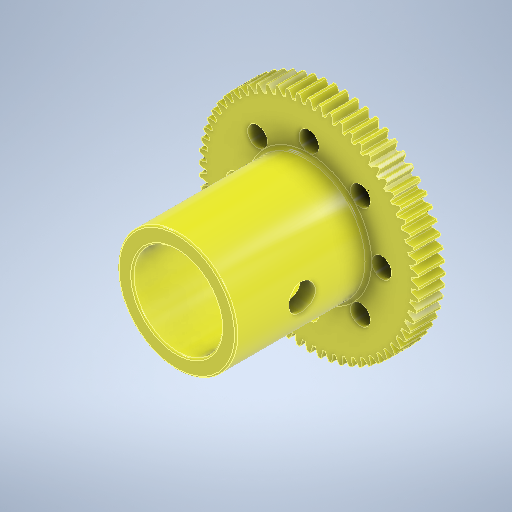
# Autodesk Inventor part: Steering Gear
Saved by Autodesk Inventor 2025.2 (Build 292293000, 293)
## iProperties
CustomPartVersion: 1
Created: 2025-02-06
Part Number: Steering Gear
Material: Steel
Document SubType Name: Modeling
Designer: eason
Categories: <?xml version="1.0" encoding="UTF-16"?> <MemberInstance><Categories><FamilyTemplate><FamilyTemplateParameter ValueType="xs:double" Id="1" ObjectReferenceKey="da_z" ObjectType="kUserParameterObject"/><FamilyTemplateParameter ValueType="xs:double" Id="2" ObjectReferenceKey="da_b" ObjectType="kUserParameterObject"/><FamilyTemplateParameter ValueType="xs:double" Id="3" ObjectReferenceKey="da_beta" ObjectType="kUserParameterObject"/><FamilyTemplateParameter ValueType="xs:double" Id="4" ObjectReferenceKey="da_da" ObjectType="kUserParameterObject"/><FamilyTemplateParameter ValueType="xs:double" Id="5" ObjectReferenceKey="da_aw" ObjectType="kUserParameterObject"/><FamilyTemplateParameter ValueType="xs:string" Id="6" ObjectReferenceKey="EAIAABAAAACIAQAAAAAAAIAAAAAAAAAA" ObjectType="83910656" SubObjectId="SurfaceGeometry"/></FamilyTemplate><ParamToTemplateMap><ParamToTemplate CategoryParameter="//CategoryParameter[@InternalName='046C89C9-8512-4d59-83FE-43B91F4F132A']" TemplateParameter="1"/><ParamToTemplate CategoryParameter="//CategoryParameter[@InternalName='2552DF32-E462-4b46-AEBF-C6C7768E72AC']" TemplateParameter="2"/><ParamToTemplate CategoryParameter="//CategoryParameter[@InternalName='C9EE641D-15FC-4fae-A226-E94C4372FDD7']" TemplateParameter="3"/><ParamToTemplate><ParamToTemplate CategoryParameter="//CategoryParameter[@InternalName='00B6519A-459B-49c7-AD84-2E56D39A5744']" ConstantValue="0.218033"/></ParamToTemplate><ParamToTemplate><ParamToTemplate CategoryParameter="//CategoryParameter[@InternalName='04B31F0E-C7A6-4894-AA32-9629BEFACF47']" ConstantValue="1.000000"/></ParamToTemplate><ParamToTemplate><ParamToTemplate CategoryParameter="//CategoryParameter[@InternalName='43CBEC2E-7847-49e7-A936-2F7889FCB2D9']" ConstantValue="0.250000"/></ParamToTemplate><ParamToTemplate><ParamToTemplate CategoryParameter="//CategoryParameter[@InternalName='B1EFC894-105D-4ebd-86BF-FA20ED196853']" ConstantValue="0.350000"/></ParamToTemplate><ParamToTemplate><ParamToTemplate CategoryParameter="//CategoryParameter[@InternalName='51175063-3D10-4879-93E8-6246FE8B403D']" ConstantValue="2060000000.000000"/></ParamToTemplate><ParamToTemplate><ParamToTemplate CategoryParameter="//CategoryParameter[@InternalName='A3A52E27-4454-46a9-B0BD-C932399B70AF']" ConstantValue="0.300000"/></ParamToTemplate><ParamToTemplate><ParamToTemplate CategoryParameter="//CategoryParameter[@InternalName='91B76062-C214-41d9-B1B9-14D2AB99603D']" ConstantValue="0.100000"/></ParamToTemplate><ParamToTemplate><ParamToTemplate CategoryParameter="//CategoryParameter[@InternalName='374E806E-8B8A-4dda-A9AA-1039D6500AD2']" ConstantValue="10.000000"/></ParamToTemplate><ParamToTemplate><ParamToTemplate CategoryParameter="//CategoryParameter[@InternalName='2D373A89-B862-43d6-8D0B-0CBF12AB9F6C']" ConstantValue="0.349066"/></ParamToTemplate><ParamToTemplate CategoryParameter="//CategoryParameter[@InternalName='37777632-D6A2-4fac-9D53-DB8ACD95C989']" TemplateParameter="4"/><ParamToTemplate CategoryParameter="//CategoryParameter[@InternalName='FD1017F1-B727-4f7e-9707-0F86F1FF9423']" TemplateParameter="5"/><ParamToTemplate><ParamToTemplate CategoryParameter="//CategoryParameter[@InternalName='9E1B4470-B2D3-4ff1-B813-535BB4CDF51A']" ConstantValue="3520000.000000"/></ParamToTemplate><ParamToTemplate><ParamToTemplate CategoryParameter="//CategoryParameter[@InternalName='F8452263-BFF6-458c-9FB1-07C4B99E95CD']" ConstantValue="11400000.000000"/></ParamToTemplate><ParamToTemplate><ParamToTemplate CategoryParameter="//CategoryParameter[@InternalName='3E3BB259-FD49-497f-8171-6EBC954A3479']" ConstantValue="2.000000"/></ParamToTemplate><ParamToTemplate CategoryParameter="//CategoryParameter[@InternalName='27C3BAF2-7550-4e4b-AE2C-0DB134B7D9B7']" TemplateParameter="6"/></ParamToTemplateMap><Category DisplayName="Gear" InternalName="DC85795E-93AB-48d5-8EEE-5A27447B64BD" Mnemonic="Gear"><CategoryParameter DisplayName="z" InternalName="046C89C9-8512-4d59-83FE-43B91F4F132A" Mnemonic="z"/><CategoryParameter DisplayName="b" InternalName="2552DF32-E462-4b46-AEBF-C6C7768E72AC" Mnemonic="b"/><CategoryParameter DisplayName="||b|" InternalName="C9EE641D-15FC-4fae-A226-E94C4372FDD7" Mnemonic="beta"/><CategoryParameter DisplayName="x" InternalName="00B6519A-459B-49c7-AD84-2E56D39A5744" Mnemonic="x"/><CategoryParameter DisplayName="a*" InternalName="04B31F0E-C7A6-4894-AA32-9629BEFACF47" Mnemonic="a"/><CategoryParameter DisplayName="c*" InternalName="43CBEC2E-7847-49e7-A936-2F7889FCB2D9" Mnemonic="c"/><CategoryParameter DisplayName="r|.f|*" InternalName="B1EFC894-105D-4ebd-86BF-FA20ED196853" Mnemonic="rf"/><CategoryParameter DisplayName="E" InternalName="51175063-3D10-4879-93E8-6246FE8B403D" Mnemonic="E"/><CategoryParameter DisplayName="||m|" InternalName="A3A52E27-4454-46a9-B0BD-C932399B70AF" Mnemonic="mi"/><Category DisplayName="SpurGear" InternalName="26C5A22E-A91E-4dfd-A3B3-23CCAFAE1764" Mnemonic="SpurGear"><CategoryParameter DisplayName="m" InternalName="91B76062-C214-41d9-B1B9-14D2AB99603D" Mnemonic="m"/><CategoryParameter DisplayName="P" InternalName="374E806E-8B8A-4dda-A9AA-1039D6500AD2" Mnemonic="PP"/><CategoryParameter DisplayName="||a|" InternalName="2D373A89-B862-43d6-8D0B-0CBF12AB9F6C" Mnemonic="alpha"/><CategoryParameter DisplayName="d|.a|" InternalName="37777632-D6A2-4fac-9D53-DB8ACD95C989" Mnemonic="da"/><CategoryParameter DisplayName="a|.w|" InternalName="FD1017F1-B727-4f7e-9707-0F86F1FF9423" Mnemonic="aw"/><CategoryParameter DisplayName="||s||.Flim|" InternalName="9E1B4470-B2D3-4ff1-B813-535BB4CDF51A" Mnemonic="sFlim"/><CategoryParameter DisplayName="||s||.Hlim|" InternalName="F8452263-BFF6-458c-9FB1-07C4B99E95CD" Mnemonic="sHlim"/><CategoryParameter DisplayName="type" InternalName="3E3BB259-FD49-497f-8171-6EBC954A3479" Mnemonic="type"/><CategoryParameter DisplayName="PitchDiameter" InternalName="27C3BAF2-7550-4e4b-AE2C-0DB134B7D9B7" Mnemonic="IDS_PITCHDIAM"/></Category></Category></Categories></MemberInstance>
Density: 1 g/cm^3
Appearance: Yellow
Author: eason
Autodesk Inventor part; units mm, degrees
sketch "Sketch1" plane through (0, 0, 0) normal (0, 0, 1) x (1, 0, 0)
  circle A0 centre (0, 0) radius 33.2138
  dimension "d0" = 66.4276
  constraints: 1 centre point
  measures "d0" diameter of A0
extrude "Extrusion1" add sketch "Sketch1" along normal blind 8
ref_plane "Work Plane2" through (0, 0, 4) normal (0, 0, 1) x (1, 0, 0)
sketch "Sketch2" plane through (0, 0, 0) normal (0, 0, -1) x (-1, 0, 0)
  circle A0 centre (0, 0) radius 33.2138 projected
  circle A1 centre (0, 0) radius 32
  dimension "d3" = 64
  constraints: 1 centre point, 1 coincident
  measures "d3" diameter of A1
surface extrude "Pitch Diameter" sketch "Sketch2" against normal through all shown no curves A1
ref_plane "Work Plane8" through (0, 0, 0) normal (0.9987955, 0.0490677, 0) x (0, 0, 1)
ref_plane "Work Plane9" through (0, 0, 0) normal (1, 0, 0) x (0, 1, 0)
spur gear teeth "Spur Gear" teeth 64 pitch diameter 64 tip diameter 66.4276 root diameter 61.9361 face width 8 start plane through (0, 0, 0) normal (0, 0, -1) x (-1, 0, 0)
sketch "Sketch3" plane through (0, 0, 8) normal (0, 0, 1) x (1, 0, 0)
  circle A0 centre (0, 0) radius 18
  circle A1 centre (0, 0) radius 13.4
  circle A2 centre (0, 0) radius 3
  dimension "d49" = 36
  dimension "d50" = 26.8
  dimension "d51" = 6
  constraints: 3 centre point, 3 coincident
  measures "d49" diameter of A0
  measures "d50" diameter of A1
  measures "d51" diameter of A2
extrude "Extrusion3" add sketch "Sketch3" along normal blind 40 contours A0
ref_plane "Work Plane11" through (18, 0, 8) normal (1, 0, 0) x (0, 1, 0)
sketch "Sketch4" plane through (18, 0, 8) normal (1, 0, 0) x (0, 1, 0)
  circle A0 centre (0, 20) radius 4
  line L0 (0, -17.6) -> (0, 49.6) projected
  line L1 (18, 40) -> (-18, 40) projected
  point P0 (0, -8)
  dimension "d56" = 8
  dimension "d57" = 20
  constraints: 1 centre point, 1 point on line
  measures "d56" diameter of A0
  measures "d57" distance from line of L1 A0.centre
extrude "Extrusion4" cut sketch "Sketch4" against normal through all
fillet "Fillet1" radius 0.5 2 edges at (-13.4, 0, 48) (-18, 0, 48)
fillet "Fillet2" radius 1 1 edges at (-18, 0, 8)
sketch "Sketch9" plane through (0, 0, 0) normal (0, 0, -1) x (-1, 0, 0)
  circle A0 centre (0, 0) radius 2 construction
  circle A1 centre (0, 0) radius 5
  circle A2 centre (-3.5, 0) radius 1.5
  line L0 (46.4993, 0) -> (-46.4993, 0) projected
  circle A3 centre (0, -3.5) radius 1.5
  circle A4 centre (3.5, 0) radius 1.5
  circle A5 centre (0, 3.5) radius 1.5
  line L1 (3.5, -1.5) -> (2, -1.5)
  line L2 (1.5, -3.5) -> (1.5, -2)
  arc A6 (2, -1.5) -> (1.5, -2) centre (2, -2) ccw
  line L3 (3.5, 1.5) -> (2, 1.5)
  arc A7 (1.5, 2) -> (2, 1.5) centre (2, 2) ccw
  line L4 (1.5, 3.5) -> (1.5, 2)
  line L5 (-1.5, 3.5) -> (-1.5, 2)
  arc A8 (-2, 1.5) -> (-1.5, 2) centre (-2, 2) ccw
  line L6 (-3.5, 1.5) -> (-2, 1.5)
  line L7 (-3.5, -1.5) -> (-2, -1.5)
  arc A9 (-1.5, -2) -> (-2, -1.5) centre (-2, -2) ccw
  line L8 (-1.5, -3.5) -> (-1.5, -2)
  point P0 (1.5, 3.5)
  dimension "d91" = 10
  dimension "d99" = 360
  dimension "d118" = 3
  dimension "d119" = 0.5
  dimension "d122" = 360
  constraints: 16 end point, 8 centre point, 8 point on circle, 4 tangent, 2 coincident, 2 horizontal, 1 perpendicular, 1 point on line, 1 vertical, 48 other
  measures "d91" diameter of A1
  measures "d118" radial gap between concentric circles of A1 A0
  measures "d119" radius of A6
extrude "Extrusion9" cut sketch "Sketch9" against normal up to surface (8 mm away) contours A4 L0 | L0 A4 | A5 | A3 | A4 L1 A6 L2 A3 L8 A9 L7 A2 L0 | L0 A2 L6 A8 L5 A5 L4 A7 L3 A4 | L0 A2 | A2 L0
sketch "Sketch11" plane through (0, 0, 0) normal (0, 0, -1) x (-1, 0, 0)
  circle A0 centre (0, 0) radius 19 projected
  circle A1 centre (0, 0) radius 25
  circle A2 centre (0, -22) radius 3
  line L0 (0, -46.4993) -> (0, 46.4993) projected
  circle A3 centre (15.5563, -15.5563) radius 3
  circle A4 centre (22, 0) radius 3
  circle A5 centre (15.5563, 15.5563) radius 3
  circle A6 centre (0, 22) radius 3
  circle A7 centre (-15.5563, 15.5563) radius 3
  circle A8 centre (-22, 0) radius 3
  circle A9 centre (-15.5563, -15.5563) radius 3
  dimension "d111" = 6
  dimension "d114" = 360
  constraints: 9 centre point, 2 tangent, 1 coincident, 1 point on line, 17 other
  measures "d111" radial gap between concentric circles of A0 A1
extrude "Extrusion11" cut sketch "Sketch11" against normal up to surface (8 mm away) contours A4 | A5 | A3 | A6 L0 | L0 A6 | L0 A2 | A2 L0 | A7 | A9 | A8
fillet "Fillet5" radius 0.5 32 edges at (1.6464, 1.6464, 8) (2.75, 1.5, 8) (5, 0, 8) (2.75, -1.5, 8) (1.6464, -1.6464, 8) (1.5, -2.75, 8) (0, -5, 8) (-1.5, -2.75, 8) (-1.6464, -1.6464, 8) (-2.75, -1.5, 8) (-5, 0, 8) (-2.75, 1.5, 8) (-1.6464, 1.6464, 8) (-1.5, 2.75, 8) (0, 5, 8) (1.5, 2.75, 8) (0, 5, 0) (-1.5, 2.75, 0) (-1.6464, 1.6464, 0) (-2.75, 1.5, 0) (-5, 0, 0) (-2.75, -1.5, 0) (-1.6464, -1.6464, 0) (-1.5, -2.75, 0) (0, -5, 0) (1.5, -2.75, 0) (1.6464, -1.6464, 0) (2.75, -1.5, 0) (5, 0, 0) (2.75, 1.5, 0) (1.6464, 1.6464, 0) (1.5, 2.75, 0)
equation "\"d0\" = da_da"
equation "\"d1\" = da_b"
equation "\"d3\" = da_d"
equation "\"d16\" = da_aw"
equation "\"d43\" = da_aw"
equation "\"d46\" = da_aw"
equation "\"da_da\" = 66.427598"
equation "\"da_b\" = 8"
equation "\"da_d\" = 64"
equation "\"da_aw\" = 40.213799"
body "Solid1"
body "Srf1"
